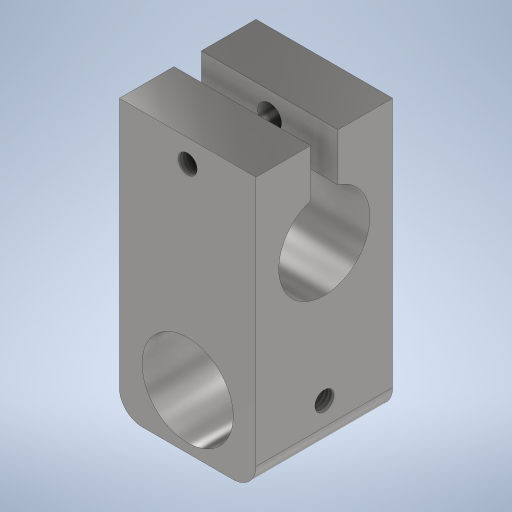
# Autodesk Inventor part: Verbindung
Saved by Autodesk Inventor 2024.4 (Build 284460000, 460)
## iProperties
Created: 2026-01-20
Part Number: Verbindung
Material: Edelstahl
Description: Verbindung
Document SubType Name: Modeling
Designer: Philf
Density: 8 g/cm^3
Appearance: Halbpoliert
Mass: 259.413 g
Surface Area: 118.776 cm^2
Volume: 32.4266 cm^3
Masse[kg]: 0,0000 kg
Autodesk Inventor part; units mm, degrees
ref_plane "YZ Plane" through (0, 0, 0) normal (1, 0, 0) x (0, 1, 0)
ref_plane "XZ Plane" through (0, 0, 0) normal (0, 1, 0) x (-1, 0, 0)
ref_plane "XY Plane" through (0, 0, 0) normal (0, 0, 1) x (1, 0, 0)
sketch "Skizze1" plane through (0, 0, 0) normal (1, 0, 0) x (0, 1, 0)
  circle A0 centre (0, 0) radius 10
  line L0 (15, 0) -> (15, -40)
  line L1 (15, -40) -> (-15, -40)
  line L2 (-15, -40) -> (-15, 0)
  line L3 (15, 0) -> (15, 20)
  line L4 (15, 20) -> (-15, 20)
  line L5 (-15, 20) -> (-15, 0)
  dimension "d0" = 20
  dimension "d2" = 40
  dimension "d3" = 30
  dimension "d4" = 90
  dimension "d40" = 20
  constraints: 12 end point, 2 perpendicular, 2 vertical, 1 centre point, 1 coincident, 1 horizontal
  measures "d0" diameter of A0
  measures "d2" distance of L0.start L0.end
  measures "d3" distance of L0.end L1.end
  measures "d4" angle of L0 L1
  measures "d40" distance of L0.start L3.end
extrude "Extrusion1" add sketch "Skizze1" along normal blind 30
sketch "Skizze3" plane through (30, 0, 0) normal (1, 0, 0) x (0, 0, -1)
  line L0 (0, 0) -> (-20, 0)
  line L1 (-20, 0) -> (-20, 3)
  line L2 (-20, 3) -> (0, 3)
  line L3 (0, 3) -> (0, 0)
  line L4 (0, 0) -> (-20, 0)
  line L5 (-20, 0) -> (-20, -3)
  line L6 (-20, -3) -> (0, -3)
  line L7 (0, -3) -> (0, 0)
  dimension "d7" = 20
  dimension "d8" = 3
  dimension "d9" = 3
  constraints: 16 end point, 4 parallel, 2 horizontal, 2 perpendicular, 1 point on line
  measures "d7" distance of L1.end L2.end
  measures "d8" distance of L0.end L1.end
  measures "d9" distance of L5.end L4.end
extrude "Extrusion2" cut sketch "Skizze3" against normal through all
sketch "Skizze6" plane through (0, 0, 0) normal (-1, 0, 0) x (0, 0, 1)
  arc A0 (9.5394, 3) -> (9.5394, -3) centre (0, 0) ccw projected
  line L0 (0, 0) -> (-30, 0)
  dimension "d31" = 30
  constraints: 2 end point, 1 horizontal
  measures "d31" distance of L0.start L0.end
hole "Bohrung3" at (0, 0, -30) direction (1, 0, 0) diameter 4.134 end through all thread size "M5x0.8" class "6H" standard "ISO Metric profile"
fillet "Rundung1" radius 5 2 edges at (0, 0, -40) (30, 0, -40)
sketch "Skizze9" plane through (0, 15, 20) normal (0, 1, 0) x (1, 0, 0)
  line L0 (30, 47.933) -> (0, 47.933) projected
  line L1 (5, 60) -> (25, 60) projected
  line L2 (15, 60) -> (15, 48)
  circle A0 centre (15, 48) radius 10
  point P0 (0, 20)
  dimension "d79" = 12
  dimension "d80" = 20
  constraints: 2 end point, 1 centre point, 1 coincident, 1 midpoint, 1 perpendicular
  measures "d79" distance of L2.start L2.end
  measures "d80" diameter of A0
extrude "Extrusion4" cut sketch "Skizze9" against normal through all
sketch "Skizze10" plane through (0, 15, 20) normal (0, 1, 0) x (1, 0, 0)
  line L0 (0, 0) -> (30, 0) projected
  line L1 (15, 0) -> (15, 5)
  point P0 (0, 20)
  dimension "d55" = 5
  constraints: 2 end point, 1 midpoint, 1 vertical
  measures "d55" distance of L1.start L1.end
hole "Bohrung5" at (15, 15, 15) direction (0, -1, 0) diameter 5.2 depth 15 tip angle 118
sketch "Skizze12" plane through (0, -15, 20) normal (0, -1, 0) x (1, 0, 0)
  circle A0 centre (15, -5) radius 2.6 projected
  line L0 (15, -5) -> (15, -13.3811)
  circle A1 centre (15, -5) radius 2.5
  point P0 (0, -20)
  dimension "d71" = 5
  constraints: 2 end point, 1 centre point, 1 coincident, 1 vertical
  measures "d71" diameter of A1
hole "Bohrung7" at (15, -15, 15) direction (0, 1, 0) diameter 4.134 end through all thread size "M5x0.8" class "6H" standard "ISO Metric profile"
